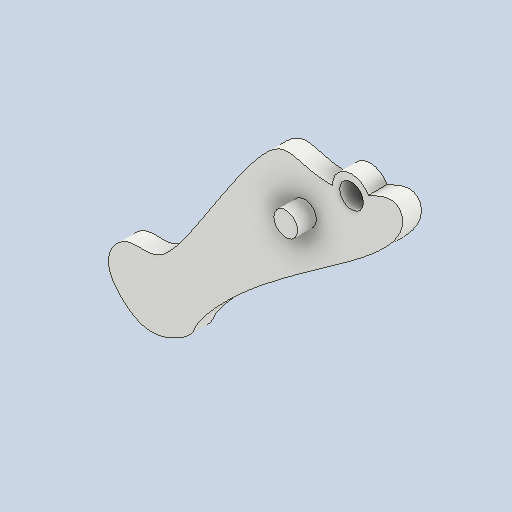
# Autodesk Inventor part: Component36
Saved by Autodesk Inventor 2022 (Build 260153000, 153)
## iProperties
Created: 2022-01-29
Part Number: Component36
Material: Generic
Document SubType Name: Modeling
Designer: Administrator
Density: 1 g/cm^3
Appearance: Default
Title: Component36
Author: Administrator
Autodesk Inventor part; units mm, degrees
ref_plane "YZ Plane" through (0, 0, 0) normal (1, 0, 0) x (0, 1, 0)
ref_plane "XZ Plane" through (0, 0, 0) normal (0, 1, 0) x (-1, 0, 0)
ref_plane "XY Plane" through (0, 0, 0) normal (0, 0, 1) x (1, 0, 0)
sketch "Sketch2" plane through (0, 0, 0) normal (0, 0, 1) x (1, 0, 0)
  circle A0 centre (17.7379, 16.3243) radius 3.175
  circle A1 centre (30.3017, 26.5478) radius 3.175
  spline S0 degree 5 poles (34.7936, 28.9205) (35.4776, 29.2207) (36.9446, 29.8791) (39.0373, 30.7866) (41.4555, 31.37) (43.7325, 30.0595) (44.4715, 26.9304) (42.8712, 22.916) (38.868, 18.2758) (32.7045, 13.1811) (24.9408, 7.6246) (16.3247, 1.6163) (7.6991, -4.7901) (-0.0485, -11.2901) (-6.1887, -17.4473) (-9.972, -22.0858) (-11.4619, -24.5671) (-11.8227, -25.7711) (-12.3858, -26.7842) (-14.1072, -28.3535) (-17.0055, -30.1951) (-20.6245, -31.6085) (-24.3173, -31.8446) (-27.6527, -30.6485) (-30.5676, -28.4364) (-32.9706, -25.7165) (-34.7172, -22.9869) (-34.8766, -19.7524) (-33.3664, -16.4658) (-30.8038, -14.1275) (-27.9175, -13.412) (-25.0571, -13.7698) (-22.1428, -13.6949) (-18.948, -11.7196) (-15.2613, -7.1808) (-11.1306, -1.126) (-6.7282, 5.6796) (-2.3012, 12.4377) (1.8897, 18.4958) (5.6272, 23.3313) (8.1618, 25.9625) (9.8273, 27.1974) (10.8678, 27.7176) (11.3773, 27.9076) (11.8868, 28.0977) (12.8844, 28.3377) (14.3572, 28.3122) (16.4933, 27.7076) (19.355, 26.8782) (22.0381, 26.4642) (24.0247, 26.3927) (25.1028, 26.423) (25.2232, 26.4273) knots 0.137303 0.137303 0.137303 0.137303 0.137303 0.137303 0.155556 0.177778 0.2 0.222222 0.244444 0.266667 0.288889 0.311111 0.333333 0.355556 0.377778 0.4 0.422222 0.444444 0.466667 0.488889 0.511111 0.533333 0.555556 0.577778 0.6 0.622222 0.644444 0.666667 0.688889 0.711111 0.733333 0.755556 0.777778 0.8 0.822222 0.844444 0.866667 0.888889 0.911111 0.933333 0.955556 0.977778 1 1 1 1 1 1.022222 1.044444 1.066667 1.088889 1.091674 1.091674 1.091674 1.091674 1.091674 1.091674 weights 1 1 1 1 1 1 1 1 1 1 1 1 1 1 1 1 1 1 1 1 1 1 1 1 1 1 1 1 1 1 1 1 1 1 1 1 1 1 1 1 1 1 1 1 1 1 1 1 1 1 1 1 1
  arc A2 (34.7936, 28.9205) -> (25.2232, 26.4273) centre (30.3017, 26.5478) ccw
  point P0 (0, 0)
  constraints: 3 centre point, 2 point on circle, 2 other
extrude "Extrusion1" add sketch "Sketch2" against normal blind 5 contours A0 | S0 A2
extrude "Extrusion2" add sketch "Sketch2" along normal blind 5 contours A0
body "Solid1"
